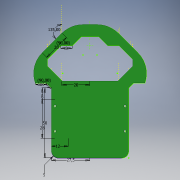
# Autodesk Inventor part: mainpcb
Saved by Autodesk Inventor 2016 (Build 200138000, 138)
## iProperties
Created: 2017-05-27
Part Number: mainpcb
Material: Ogólny
Document SubType Name: Modeling
Designer: Karol
Density: 1 g/cm^3
Appearance: Smooth - Dark Forest Green
Author: Karol
Autodesk Inventor part; units mm, degrees
ref_plane "YZ Plane" through (0, 0, 0) normal (1, 0, 0) x (0, 1, 0)
ref_plane "XZ Plane" through (0, 0, 0) normal (0, 1, 0) x (-1, 0, 0)
ref_plane "XY Plane" through (0, 0, 0) normal (0, 0, 1) x (1, 0, 0)
sketch "Sketch1" plane through (0, 0, 0) normal (0, 1, 0) x (-1, 0, 0)
  line L0 (0, 0) -> (0, 22.5)
  line L1 (5, 27.5) -> (50, 27.5)
  arc A0 (5, 27.5) -> (0, 22.5) centre (5, 22.5) ccw
  arc A1 (95.1955, 5) -> (89.1353, 20) centre (73.6017, 5) ccw
  line L2 (89.1353, 20) -> (74.9931, 34.1421)
  line L3 (89.1353, 20) -> (109.1353, 20) construction
  line L4 (71.2668, 30.4158) -> (81.2668, 30.4158) construction
  line L5 (71.4576, 30.6066) -> (81.4576, 30.6066) construction
  line L6 (26, 0) -> (39.959, 0)
  line L7 (95.1955, 5) -> (95.1955, 0)
  line L8 (0, 0) -> (0, -22.5)
  line L9 (5, -27.5) -> (50, -27.5)
  arc A2 (0, -22.5) -> (5, -27.5) centre (5, -22.5) ccw
  line L10 (89.1353, 20) -> (109.1353, 20) construction
  line L11 (80.3871, 20) -> (92.3871, 20) construction
  line L12 (80.3871, 20) -> (92.3871, 20) construction
  line L13 (71.7845, 29.1924) -> (83.2845, 29.1924) construction
  line L14 (80.2613, 15.3464) -> (87.6044, 15.3464) construction
  line L15 (80.2613, 20.8464) -> (93.9162, 20.8464) construction
  line L16 (80.2613, 20.8464) -> (92.6179, 20.8464) construction
  line L17 (50, 27.5) -> (53.5355, 31.0355)
  line L18 (54.8259, 20.1488) -> (64.5921, 20.1488) construction
  line L19 (50, 27.5) -> (65, 27.5) construction
  line L20 (50, 27.5) -> (65, 27.5) construction
  line L21 (54.8259, 20.1488) -> (64.5921, 20.1488) construction
  line L22 (54.8259, 20.1488) -> (67.5921, 20.1488) construction
  line L23 (54.8259, 20.1488) -> (68.169, 20.1488) construction
  line L24 (53.5355, 31.0355) -> (53.5355, 39.0355)
  line L25 (53.5355, 31.0355) -> (61.5355, 31.0355) construction
  arc A3 (74.9931, 34.1421) -> (53.5355, 39.0355) centre (60.372, 19.521) ccw
  line L26 (70.4238, 30.6838) -> (80.2613, 20.8464)
  line L27 (80.2613, 20.8464) -> (80.2613, 12.8464)
  line L28 (80.2613, 20.8464) -> (88.2613, 20.8464) construction
  line L29 (80.2613, 12.8464) -> (88.6327, 12.8464) construction
  line L30 (80.2613, 12.8464) -> (86.6252, 6.4816)
  line L31 (86.6252, 6.4816) -> (86.6252, 0)
  arc A4 (89.1353, -20) -> (95.1955, -5) centre (73.6017, -5) ccw
  line L32 (89.1353, -20) -> (74.9931, -34.1421)
  line L33 (71.2668, -30.4158) -> (81.2668, -30.4158) construction
  line L34 (71.4576, -30.6066) -> (81.4576, -30.6066) construction
  line L35 (95.1955, -5) -> (95.1955, 0)
  line L36 (80.3871, -20) -> (92.3871, -20) construction
  line L37 (80.3871, -20) -> (92.3871, -20) construction
  line L38 (71.7845, -29.1924) -> (83.2845, -29.1924) construction
  line L39 (80.2613, -15.3464) -> (87.6044, -15.3464) construction
  line L40 (80.2613, -20.8464) -> (93.9162, -20.8464) construction
  line L41 (80.2613, -20.8464) -> (92.6179, -20.8464) construction
  line L42 (50, -27.5) -> (53.5355, -31.0355)
  line L43 (54.8259, -20.1488) -> (64.5921, -20.1488) construction
  line L44 (54.8259, -20.1488) -> (67.5921, -20.1488) construction
  line L45 (54.8259, -20.1488) -> (68.169, -20.1488) construction
  line L46 (50, -27.5) -> (65, -27.5) construction
  line L47 (50, -27.5) -> (65, -27.5) construction
  line L48 (53.5355, -31.0355) -> (53.5355, -39.0355)
  line L49 (53.5355, -31.0355) -> (61.5355, -31.0355) construction
  arc A5 (53.5355, -39.0355) -> (74.9931, -34.1421) centre (60.372, -19.521) ccw
  line L50 (70.4238, -30.6838) -> (80.2613, -20.8464)
  line L51 (80.2613, -20.8464) -> (80.2613, -12.8464)
  line L52 (80.2613, -20.8464) -> (88.2613, -20.8464) construction
  line L53 (80.2613, -12.8464) -> (88.6327, -12.8464) construction
  line L54 (80.2613, -12.8464) -> (86.6252, -6.4816)
  line L55 (86.6252, -6.4816) -> (86.6252, 0)
  line L56 (54.8259, 0) -> (54.8259, 20)
  line L57 (54.8259, 20) -> (65.5088, 30.6838)
  line L58 (65.5088, 30.6838) -> (70.4238, 30.6838)
  line L59 (54.8259, -20.1488) -> (64.5921, -20.1488) construction
  line L60 (54.8259, -20.1488) -> (64.5921, -20.1488) construction
  line L61 (54.8259, -20.1488) -> (67.5921, -20.1488) construction
  line L62 (54.8259, -20.1488) -> (68.169, -20.1488) construction
  line L63 (54.8259, 0) -> (54.8259, -20)
  line L64 (54.8259, -20) -> (65.5088, -30.6838)
  line L65 (65.5088, -30.6838) -> (70.4238, -30.6838)
  point P0 (0, 27.5)
  point P1 (80, 0)
  point P2 (42, 25)
  point P3 (14, 25)
  point P4 (14, 15.5)
  point P5 (37, 25)
  point P6 (19, 25)
  point P7 (0, -27.5)
  point P8 (42, -25)
  point P9 (14, -25)
  point P10 (14, -15.5)
  point P11 (37, -25)
  point P12 (19, -25)
  dimension "d2" = 27.5
  dimension "d3" = 50
  dimension "d19" = 5
  dimension "d42" = 8
  dimension "d43" = 28
  dimension "d45" = 12
  dimension "d73" = 20
  dimension "d74" = 135
  dimension "d105" = 5
  dimension "d118" = 8
  dimension "d119" = 90
  dimension "d120" = 8
  dimension "d121" = 90
  dimension "d123" = 20
  constraints: 132 end point, 47 symmetric about line, 15 horizontal, 12 point on circle, 6 centre point, 5 vertical, 4 point on line, 3 equal length, 3 tangent, 1 perpendicular, 3 other
  measures "d2" distance of L0.start point (0, 27.5)
  measures "d3" distance of point (0, 27.5) L1.end
  measures "d19" radius of A0
  measures "d42" horizontal distance of L1.end point (42, 25)
  measures "d43" distance of point (14, 25) point (42, 25)
  measures "d45" distance from line of L1 point (14, 15.5)
  measures "d73" distance of L2.start L2.end
  measures "d74" angle of L3 L2
  measures "d105" distance of L1.end L17.end
  measures "d118" distance of L17.end L24.end
  measures "d119" angle of L25 L24
  measures "d120" distance of L15.start L27.end
  measures "d121" angle of L27 L28
  measures "d123" distance of L56.start L56.end
extrude "Extrusion1" add sketch "Sketch1" along normal blind 1.4
hole "Hole1" at (-37, 0, 25) at (-19, 0, 25) at (-37, 0, -25) at (-19, 0, -25) direction (0, 1, 0) diameter 2 depth 2 tip angle 118
hole "Hole3" at (-14, 0, 15.5) direction (0, 1, 0) diameter 0.1 depth 8 tip angle 118
body "Solid1"
